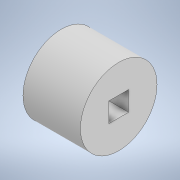
# Autodesk Inventor part: 220218 Large Rod Attachment (plain - remastered - adjusted 0.02 inch)
Saved by Autodesk Inventor 2022 (Build 260153000, 153)
## iProperties
Created: 2022-01-27
Part Number: 220218 Large Rod Attachment (plain - remastered - adjusted 0.02 inch)
Material: Generic
Document SubType Name: Modeling
Designer: josephinew
Density: 1 g/cm^3
Appearance: Default
Author: josephinew
Autodesk Inventor part; units mm, degrees
ref_plane "YZ Plane" through (0, 0, 0) normal (1, 0, 0) x (0, 1, 0)
ref_plane "XZ Plane" through (0, 0, 0) normal (0, 1, 0) x (-1, 0, 0)
ref_plane "XY Plane" through (0, 0, 0) normal (0, 0, 1) x (1, 0, 0)
sketch "Sketch1" plane through (0, 0, 0) normal (1, 0, 0) x (0, 1, 0)
  circle A0 centre (0, 0) radius 50.8
  line L0 (13.081, 13.081) -> (-13.081, 13.081)
  line L1 (-13.081, 13.081) -> (-13.081, -13.081)
  line L2 (-13.081, -13.081) -> (13.081, -13.081)
  line L3 (13.081, -13.081) -> (13.081, 13.081)
  line L4 (13.081, 0) -> (-13.081, 0)
  line L5 (0, 13.081) -> (0, 0)
  dimension "d0" = 101.6
  dimension "d1" = 26.162
  dimension "d2" = 26.162
  constraints: 12 end point, 4 midpoint, 2 parallel, 1 centre point, 1 coincident, 1 horizontal, 1 perpendicular, 1 vertical
  measures "d0" diameter of A0
  measures "d1" distance of L2.end L1.end
  measures "d2" distance of L1.end L0.end
extrude "Extrusion1" add sketch "Sketch1" along normal blind 76.2
body "Solid1"
